Autodesk Fusion 360 part; units mm, degrees
(part 2 of 3)
  line L1099 (31, -19.3397) -> (16, -10.6795)
  line L1100 (63, -19.3397) -> (48, -10.6795)
  line L1101 (31, -19.3397) -> (16, -10.6795)
  line L1102 (-33, -19.3397) -> (-48, -10.6795)
  line L1103 (-1, -36.6603) -> (-1, -19.3397)
  line L1104 (-33, -19.3397) -> (-48, -10.6795)
  line L1105 (-1, -19.3397) -> (-16, -10.6795)
  line L1106 (-33, -19.3397) -> (-48, -10.6795)
  line L1107 (63, -19.3397) -> (48, -10.6795)
  line L1108 (16, -10.6795) -> (1, -19.3397)
  line L1109 (48, -10.6795) -> (33, -19.3397)
  line L1110 (-48, -10.6795) -> (-63, -19.3397)
  line L1111 (48, -10.6795) -> (33, -19.3397)
  line L1112 (-48, -10.6795) -> (-63, -19.3397)
  line L1113 (-33, -36.6603) -> (-33, -19.3397)
  line L1114 (-33, -19.3397) -> (-48, -10.6795)
  line L1115 (-48, -10.6795) -> (-63, -19.3397)
  line L1116 (-31, -19.3397) -> (-31, -36.6603)
  line L1117 (31, -19.3397) -> (16, -10.6795)
  line L1118 (31, -19.3397) -> (16, -10.6795)
  line L1119 (63, -19.3397) -> (48, -10.6795)
  line L1120 (-1, -36.6603) -> (-1, -19.3397)
  line L1121 (48, -10.6795) -> (33, -19.3397)
  line L1122 (48, -10.6795) -> (33, -19.3397)
  line L1123 (-1, -19.3397) -> (-16, -10.6795)
  line L1124 (-48, -10.6795) -> (-63, -19.3397)
  line L1125 (-1, -19.3397) -> (-16, -10.6795)
  line L1126 (-48, -10.6795) -> (-63, -19.3397)
  line L1127 (-1, -36.6603) -> (-1, -19.3397)
  line L1128 (-1, -19.3397) -> (-16, -10.6795)
  line L1129 (-1, -36.6603) -> (-1, -19.3397)
  line L1130 (31, -19.3397) -> (16, -10.6795)
  line L1131 (-1, -19.3397) -> (-16, -10.6795)
  line L1132 (-16, -10.6795) -> (-31, -19.3397)
  line L1133 (-16, -10.6795) -> (-31, -19.3397)
  line L1134 (-33, -36.6603) -> (-33, -19.3397)
  line L1135 (1, -19.3397) -> (1, -36.6603)
  line L1136 (-16, -10.6795) -> (-31, -19.3397)
  line L1137 (1, -19.3397) -> (1, -36.6603)
  line L1138 (1, -19.3397) -> (1, -36.6603)
  line L1139 (-16, -10.6795) -> (-31, -19.3397)
  line L1140 (-16, -10.6795) -> (-31, -19.3397)
  line L1141 (63, -36.6603) -> (63, -19.3397)
  line L1142 (-31, -19.3397) -> (-31, -36.6603)
  line L1143 (-16, -10.6795) -> (-31, -19.3397)
  line L1144 (31, -36.6603) -> (31, -19.3397)
  line L1145 (-16, -10.6795) -> (-31, -19.3397)
  line L1146 (-48, 10.6795) -> (-33, 19.3397)
  line L1147 (33, -19.3397) -> (33, -36.6603)
  line L1148 (32, 17.3205) -> (17, 8.6603)
  line L1149 (33, -19.3397) -> (33, -36.6603)
  line L1150 (-32, -17.3205) -> (-17, -8.6603)
  line L1151 (1, -19.3397) -> (1, -36.6603)
  line L1152 (-32, -17.3205) -> (-17, -8.6603)
  line L1153 (-63, 19.3397) -> (-48, 10.6795)
  line L1154 (31, -36.6603) -> (31, -19.3397)
  line L1155 (31, -36.6603) -> (31, -19.3397)
  line L1156 (31, -36.6603) -> (31, -19.3397)
  line L1157 (-64, 17.3205) -> (-79, 8.6603)
  line L1158 (0, 17.3205) -> (-15, 8.6603)
  line L1159 (1, -19.3397) -> (1, -36.6603)
  line L1160 (-16, -10.6795) -> (-31, -19.3397)
  line L1161 (16, 10.6795) -> (31, 19.3397)
  line L1162 (-16, -10.6795) -> (-31, -19.3397)
  line L1163 (1, -19.3397) -> (1, -36.6603)
  line L1164 (-33, -36.6603) -> (-33, -19.3397)
  line L1165 (-31, -19.3397) -> (-31, -36.6603)
  line L1166 (-16, -10.6795) -> (-31, -19.3397)
  line L1167 (32, 17.3205) -> (17, 8.6603)
  line L1168 (1, -19.3397) -> (1, -36.6603)
  line L1169 (-16, -10.6795) -> (-31, -19.3397)
  line L1170 (-16, -10.6795) -> (-31, -19.3397)
  line L1171 (33, 19.3397) -> (48, 10.6795)
  line L1172 (-64, 17.3205) -> (-79, 8.6603)
  line L1173 (48, 10.6795) -> (63, 19.3397)
  line L1174 (-16, -10.6795) -> (-31, -19.3397)
  line L1175 (-48, 10.6795) -> (-33, 19.3397)
  line L1176 (-16, -10.6795) -> (-31, -19.3397)
  line L1177 (-16, -10.6795) -> (-31, -19.3397)
  line L1178 (-16, 10.6795) -> (-1, 19.3397)
  line L1179 (32, 17.3205) -> (17, 8.6603)
  line L1180 (1, -19.3397) -> (1, -36.6603)
  line L1181 (-16, -10.6795) -> (-31, -19.3397)
  line L1182 (-16, -10.6795) -> (-31, -19.3397)
  line L1183 (32, 17.3205) -> (17, 8.6603)
  line L1184 (-31, -19.3397) -> (-31, -36.6603)
  line L1185 (48, 10.6795) -> (63, 19.3397)
  line L1186 (16, 10.6795) -> (31, 19.3397)
  line L1187 (-16, -10.6795) -> (-31, -19.3397)
  line L1188 (-33, -36.6603) -> (-33, -19.3397)
  line L1189 (-49, 8.6603) -> (-64, 17.3205)
  line L1190 (-32, -17.3205) -> (-17, -8.6603)
  line L1191 (33, -19.3397) -> (33, -36.6603)
  line L1192 (31, -36.6603) -> (31, -19.3397)
  line L1193 (-32, -17.3205) -> (-17, -8.6603)
  line L1194 (1, -19.3397) -> (1, -36.6603)
  line L1195 (-16, -10.6795) -> (-31, -19.3397)
  line L1196 (-16, -10.6795) -> (-31, -19.3397)
  line L1197 (31, -36.6603) -> (31, -19.3397)
  line L1198 (-16, -10.6795) -> (-31, -19.3397)
  line L1199 (-63, 19.3397) -> (-48, 10.6795)
  line L1200 (31, -36.6603) -> (31, -19.3397)
  line L1201 (64, 17.3205) -> (49, 8.6603)
  line L1202 (64, 17.3205) -> (49, 8.6603)
  line L1203 (-32, 17.3205) -> (-47, 8.6603)
  line L1204 (17, -8.6603) -> (32, -17.3205)
  line L1205 (-33, -36.6603) -> (-33, -19.3397)
  line L1206 (31, -36.6603) -> (31, -19.3397)
  line L1207 (-31, -19.3397) -> (-31, -36.6603)
  line L1208 (1, -19.3397) -> (1, -36.6603)
  line L1209 (-32, -17.3205) -> (-17, -8.6603)
  line L1210 (-16, -10.6795) -> (-31, -19.3397)
  line L1211 (-33, -36.6603) -> (-33, -19.3397)
  line L1212 (-33, -36.6603) -> (-33, -19.3397)
  line L1213 (-33, -36.6603) -> (-33, -19.3397)
  line L1214 (-64, 17.3205) -> (-79, 8.6603)
  line L1215 (1, -19.3397) -> (1, -36.6603)
  line L1216 (-16, -10.6795) -> (-31, -19.3397)
  line L1217 (-16, -10.6795) -> (-31, -19.3397)
  line L1218 (31, -36.6603) -> (31, -19.3397)
  line L1219 (31, -36.6603) -> (31, -19.3397)
  line L1220 (-16, -10.6795) -> (-31, -19.3397)
  line L1221 (-64, 17.3205) -> (-79, 8.6603)
  line L1222 (-31, -19.3397) -> (-31, -36.6603)
  line L1223 (47, 8.6603) -> (32, 17.3205)
  line L1224 (1, -19.3397) -> (1, -36.6603)
  line L1225 (-16, -10.6795) -> (-31, -19.3397)
  line L1226 (33, 19.3397) -> (48, 10.6795)
  line L1227 (-49, 8.6603) -> (-64, 17.3205)
  line L1228 (79, 8.6603) -> (64, 17.3205)
  line L1229 (1, -19.3397) -> (1, -36.6603)
  line L1230 (-31, -19.3397) -> (-31, -36.6603)
  line L1231 (63, -36.6603) -> (63, -19.3397)
  line L1232 (33, -19.3397) -> (33, -36.6603)
  line L1233 (79, 8.6603) -> (64, 17.3205)
  line L1234 (-49, 8.6603) -> (-64, 17.3205)
  line L1235 (-49, 8.6603) -> (-64, 17.3205)
  line L1236 (47, 8.6603) -> (32, 17.3205)
  line L1237 (-31, -19.3397) -> (-31, -36.6603)
  line L1238 (79, 8.6603) -> (64, 17.3205)
  line L1239 (79, 8.6603) -> (64, 17.3205)
  line L1240 (47, 8.6603) -> (32, 17.3205)
  line L1241 (-32, -17.3205) -> (-17, -8.6603)
  line L1242 (31, -36.6603) -> (31, -19.3397)
  line L1243 (-17, 8.6603) -> (-32, 17.3205)
  line L1244 (64, 17.3205) -> (49, 8.6603)
  line L1245 (-33, -36.6603) -> (-33, -19.3397)
  line L1246 (31, -36.6603) -> (31, -19.3397)
  line L1247 (47, 8.6603) -> (32, 17.3205)
  line L1248 (31, -36.6603) -> (31, -19.3397)
  line L1249 (-16, -10.6795) -> (-31, -19.3397)
  line L1250 (63, -36.6603) -> (63, -19.3397)
  line L1251 (1, -19.3397) -> (1, -36.6603)
  line L1252 (31, -36.6603) -> (31, -19.3397)
  line L1253 (31, -36.6603) -> (31, -19.3397)
  line L1254 (64, 17.3205) -> (49, 8.6603)
  line L1255 (-1, -19.3397) -> (-16, -10.6795)
  line L1256 (-1, -36.6603) -> (-1, -19.3397)
  line L1257 (-32, 17.3205) -> (-47, 8.6603)
  line L1258 (-31, -19.3397) -> (-31, -36.6603)
  line L1259 (15, 8.6603) -> (0, 17.3205)
  line L1260 (15, 8.6603) -> (0, 17.3205)
  line L1261 (-17, 8.6603) -> (-32, 17.3205)
  line L1262 (-1, -36.6603) -> (-1, -19.3397)
  line L1263 (-1, -19.3397) -> (-16, -10.6795)
  line L1264 (-1, -36.6603) -> (-1, -19.3397)
  line L1265 (17, -8.6603) -> (32, -17.3205)
  line L1266 (-31, 19.3397) -> (-16, 10.6795)
  line L1267 (17, -8.6603) -> (32, -17.3205)
  line L1268 (-32, 17.3205) -> (-47, 8.6603)
  line L1269 (-48, -10.6795) -> (-63, -19.3397)
  line L1270 (17, -8.6603) -> (32, -17.3205)
  line L1271 (-33, -19.3397) -> (-48, -10.6795)
  line L1272 (-33, -36.6603) -> (-33, -19.3397)
  line L1273 (-1, -36.6603) -> (-1, -19.3397)
  line L1274 (-1, -36.6603) -> (-1, -19.3397)
  line L1275 (-31, 19.3397) -> (-16, 10.6795)
  line L1276 (-17, 8.6603) -> (-32, 17.3205)
  line L1277 (17, -8.6603) -> (32, -17.3205)
  line L1278 (-1, -36.6603) -> (-1, -19.3397)
  line L1279 (-31, -19.3397) -> (-31, -36.6603)
  line L1280 (15, 8.6603) -> (0, 17.3205)
  line L1281 (1, 19.3397) -> (16, 10.6795)
  line L1282 (-17, 8.6603) -> (-32, 17.3205)
  line L1283 (-1, -19.3397) -> (-16, -10.6795)
  line L1284 (-1, -36.6603) -> (-1, -19.3397)
  line L1285 (-32, 17.3205) -> (-47, 8.6603)
  line L1286 (17, -8.6603) -> (32, -17.3205)
  line L1287 (15, 8.6603) -> (0, 17.3205)
  line L1288 (-1, -36.6603) -> (-1, -19.3397)
  line L1289 (1, 19.3397) -> (16, 10.6795)
  line L1290 (-1, -36.6603) -> (-1, -19.3397)
  line L1291 (-33, -36.6603) -> (-33, -19.3397)
  line L1292 (-33, -19.3397) -> (-48, -10.6795)
  line L1293 (-48, -10.6795) -> (-63, -19.3397)
  line L1294 (17, -8.6603) -> (32, -17.3205)
  line L1295 (-79, -8.6603) -> (-64, -17.3205)
  line L1296 (-64, -17.3205) -> (-49, -8.6603)
  line L1297 (-64, -17.3205) -> (-49, -8.6603)
  line L1298 (-15, 8.6603) -> (-15, -8.6603)
  line L1299 (-79, -8.6603) -> (-64, -17.3205)
  line L1300 (-15, 8.6603) -> (-15, -8.6603)
  line L1301 (-64, -17.3205) -> (-49, -8.6603)
  line L1302 (-79, -8.6603) -> (-64, -17.3205)
  line L1303 (-79, -8.6603) -> (-64, -17.3205)
  line L1304 (-64, -17.3205) -> (-49, -8.6603)
  line L1305 (-79, 8.6603) -> (-79, -8.6603)
  line L1306 (-79, -8.6603) -> (-64, -17.3205)
  line L1307 (-79, -8.6603) -> (-64, -17.3205)
  line L1308 (-47, 8.6603) -> (-47, -8.6603)
  line L1309 (-49, -8.6603) -> (-49, 8.6603)
  line L1310 (15, -8.6603) -> (15, 8.6603)
  line L1311 (-49, -8.6603) -> (-49, 8.6603)
  line L1312 (-15, 8.6603) -> (-15, -8.6603)
  line L1313 (-17, -8.6603) -> (-17, 8.6603)
  line L1314 (31, -36.6603) -> (31, -19.3397)
  line L1315 (1, -19.3397) -> (1, -36.6603)
  line L1316 (-15, 8.6603) -> (-15, -8.6603)
  line L1317 (1, -19.3397) -> (1, -36.6603)
  line L1318 (-33, -36.6603) -> (-33, -19.3397)
  line L1319 (-16, -10.6795) -> (-31, -19.3397)
  line L1320 (-79, 8.6603) -> (-79, -8.6603)
  line L1321 (-49, -8.6603) -> (-49, 8.6603)
  line L1322 (79, -8.6603) -> (79, 8.6603)
  line L1323 (0, -17.3205) -> (15, -8.6603)
  line L1324 (0, -17.3205) -> (15, -8.6603)
  line L1325 (0, -17.3205) -> (15, -8.6603)
  line L1326 (-31, -19.3397) -> (-31, -36.6603)
  line L1327 (0, -17.3205) -> (15, -8.6603)
  line L1328 (79, -8.6603) -> (79, 8.6603)
  line L1329 (17, 8.6603) -> (17, -8.6603)
  line L1330 (-16, 10.6795) -> (-1, 19.3397)
  line L1331 (47, -8.6603) -> (47, 8.6603)
  line L1332 (-79, 8.6603) -> (-79, -8.6603)
  line L1333 (15, -8.6603) -> (15, 8.6603)
  line L1334 (-47, 8.6603) -> (-47, -8.6603)
  line L1335 (49, 8.6603) -> (49, -8.6603)
  line L1336 (49, 8.6603) -> (49, -8.6603)
  line L1337 (0, -17.3205) -> (15, -8.6603)
  line L1338 (0, -17.3205) -> (15, -8.6603)
  line L1339 (-33, -36.6603) -> (-33, -19.3397)
  line L1340 (0, -17.3205) -> (15, -8.6603)
  line L1341 (0, -17.3205) -> (15, -8.6603)
  line L1342 (63, -36.6603) -> (63, -19.3397)
  line L1343 (-33, -36.6603) -> (-33, -19.3397)
  line L1344 (0, 17.3205) -> (-15, 8.6603)
  line L1345 (-17, -8.6603) -> (-17, 8.6603)
  line L1346 (17, 8.6603) -> (17, -8.6603)
  line L1347 (-32, -17.3205) -> (-17, -8.6603)
  line L1348 (-31, -19.3397) -> (-31, -36.6603)
  line L1349 (-16, -10.6795) -> (-31, -19.3397)
  line L1350 (0, 17.3205) -> (-15, 8.6603)
  line L1351 (-32, -17.3205) -> (-17, -8.6603)
  line L1352 (-16, -10.6795) -> (-31, -19.3397)
  line L1353 (15, -8.6603) -> (15, 8.6603)
  line L1354 (-49, -8.6603) -> (-49, 8.6603)
  line L1355 (47, -8.6603) -> (47, 8.6603)
  line L1356 (17, 8.6603) -> (17, -8.6603)
  line L1357 (-47, 8.6603) -> (-47, -8.6603)
  line L1358 (-16, -10.6795) -> (-31, -19.3397)
  line L1359 (-16, -10.6795) -> (-31, -19.3397)
  line L1360 (0, 17.3205) -> (-15, 8.6603)
  line L1361 (-17, -8.6603) -> (-17, 8.6603)
  line L1362 (-47, 8.6603) -> (-47, -8.6603)
  line L1363 (79, -8.6603) -> (79, 8.6603)
  line L1364 (-31, -19.3397) -> (-31, -36.6603)
  line L1365 (49, 8.6603) -> (49, -8.6603)
  line L1366 (-33, -36.6603) -> (-33, -19.3397)
  line L1367 (47, -8.6603) -> (47, 8.6603)
  line L1368 (-31, -19.3397) -> (-31, -36.6603)
  line L1369 (49, 8.6603) -> (49, -8.6603)
  line L1370 (15, -8.6603) -> (15, 8.6603)
  line L1371 (-31, -19.3397) -> (-31, -36.6603)
  line L1372 (-63, -36.6603) -> (-48, -45.3205)
  line L1373 (-48, -45.3205) -> (-33, -36.6603)
  line L1374 (-31, -36.6603) -> (-16, -45.3205)
  line L1375 (-16, -45.3205) -> (-1, -36.6603)
  line L1376 (1, -36.6603) -> (16, -45.3205)
  line L1377 (16, -45.3205) -> (31, -36.6603)
  line L1378 (48, -45.3205) -> (63, -36.6603)
  line L1379 (33, -36.6603) -> (48, -45.3205)
  line L1380 (-32, 73.3205) -> (-47, 64.6603)
  line L1381 (-47, 64.6603) -> (-47, 47.3397)
  line L1382 (-47, 47.3397) -> (-32, 38.6795)
  line L1383 (-32, 38.6795) -> (-17, 47.3397)
  line L1384 (-17, 47.3397) -> (-17, 64.6603)
  line L1385 (-17, 64.6603) -> (-32, 73.3205)
  line L1386 (0, 38.6795) -> (15, 47.3397)
  line L1387 (-15, 47.3397) -> (0, 38.6795)
  line L1388 (-15, 64.6603) -> (-15, 47.3397)
  line L1389 (0, 73.3205) -> (-15, 64.6603)
  line L1390 (15, 64.6603) -> (0, 73.3205)
  line L1391 (15, 47.3397) -> (15, 64.6603)
  line L1392 (47, 47.3397) -> (47, 64.6603)
  line L1393 (32, 38.6795) -> (47, 47.3397)
  line L1394 (17, 47.3397) -> (32, 38.6795)
  line L1395 (17, 64.6603) -> (17, 47.3397)
  line L1396 (32, 73.3205) -> (17, 64.6603)
  line L1397 (47, 64.6603) -> (32, 73.3205)
  circle A1 centre (0, 0) radius 62
  point P0 (32, 0)
  point P1 (32, 0)
  point P2 (32, 0)
  point P3 (32, 0)
  point P4 (32, 0)
  point P5 (32, 0)
  point P6 (-32, 0)
  point P7 (-32, 0)
  point P8 (-32, 0)
  point P9 (-32, 0)
  point P10 (-32, 0)
  point P11 (-32, 0)
  point P12 (-64, 0)
  point P13 (-64, 0)
  point P14 (-64, 0)
  point P15 (-64, 0)
  point P16 (-64, 0)
  point P17 (-64, 0)
  point P18 (64, 0)
  point P19 (64, 0)
  point P20 (64, 0)
  point P21 (64, 0)
  point P22 (64, 0)
  point P23 (64, 0)
  point P24 (-16, -28)
  point P25 (-16, -28)
  point P26 (-16, -28)
  point P27 (-16, -28)
  point P28 (-16, -28)
  point P29 (-16, -28)
  point P30 (-32, -17.3205)
  point P31 (0, -17.3205)
  point P32 (-16, -28)
  point P33 (-16, -28)
  point P34 (-16, -28)
  point P35 (-16, -28)
  point P36 (-16, -28)
  point P37 (-16, -28)
  point P38 (0, -17.3205)
  point P39 (32, -17.3205)
  point P40 (16, -28)
  point P41 (32, -17.3205)
  point P42 (16, -28)
  point P43 (16, -28)
  point P44 (16, -28)
  point P45 (16, -28)
  point P46 (16, -28)
  point P47 (16, -28)
  point P48 (16, -28)
  point P49 (16, -28)
  point P50 (16, -28)
  point P51 (16, -28)
  point P52 (0, -17.3205)
  point P53 (16, -28)
  point P54 (-49, -8.6603)
  point P55 (-49, -8.6603)
  point P56 (-64, -17.3205)
  point P57 (-47, -8.6603)
  point P58 (-47, -8.6603)
  point P59 (-48, -28)
  point P60 (-48, -28)
  point P61 (-48, -28)
  point P62 (-48, -28)
  point P63 (-48, -28)
  point P64 (-48, -28)
  point P65 (-48, -28)
  point P66 (-48, -28)
  point P67 (-48, -28)
  point P68 (-48, -28)
  point P69 (-48, -28)
  point P70 (-64, -17.3205)
  point P71 (-48, -28)
  point P72 (-32, -56)
  point P73 (-32, -56)
  point P74 (-32, -56)
  point P75 (-64, -56)
  point P76 (-32, -56)
  point P77 (-32, -56)
  point P78 (-32, -56)
  point P79 (32, -56)
  point P80 (32, -56)
  point P81 (32, -56)
  point P82 (32, -56)
  point P83 (0, -56)
  point P84 (0, -56)
  point P85 (32, -56)
  point P86 (0, -56)
  point P87 (32, -56)
  point P88 (0, -56)
  point P89 (0, -56)
  point P90 (0, -56)
  point P91 (32, -73.3205)
  point P92 (0, -73.3205)
  point P93 (-16, -84)
  point P94 (0, -73.3205)
  point P95 (16, -84)
  point P96 (16, -84)
  point P97 (16, -84)
  point P98 (16, -84)
  point P99 (-16, -84)
  point P100 (-16, -84)
  point P101 (-16, -84)
  point P102 (16, -84)
  point P103 (16, -84)
  point P104 (16, -84)
  point P105 (16, -84)
  point P106 (-16, -84)
  point P107 (-16, -84)
  point P108 (16, -84)
  point P109 (16, -84)
  point P110 (16, -84)
  point P111 (32, -73.3205)
  point P112 (-64, -56)
  point P113 (-64, -56)
  point P114 (64, -56)
  point P115 (-64, -56)
  point P116 (-16, -84)
  point P117 (-64, -56)
  point P118 (64, -56)
  point P119 (-16, -84)
  point P120 (-16, -84)
  point P121 (64, -56)
  point P122 (-16, -84)
  point P123 (-16, -84)
  point P124 (-32, -73.3205)
  point P125 (-16, -84)
  point P126 (64, -56)
  point P127 (64, -56)
  point P128 (-64, -56)
  point P129 (64, -56)
  point P130 (-49, -64.6603)
  point P131 (0, -73.3205)
  point P132 (-49, -64.6603)
  point P133 (-48, -84)
  point P134 (-48, -84)
  point P135 (-47, -64.6603)
  point P136 (-47, -64.6603)
  point P137 (-48, -84)
  point P138 (-48, -84)
  point P139 (-48, -84)
  point P140 (-48, -84)
  point P141 (-48, -84)
  point P142 (-48, -84)
  point P143 (16, -84)
  point P144 (-64, -73.3205)
  point P145 (-48, -84)
  point P146 (33, -75.3397)
  point P147 (-64, -73.3205)
  point P148 (-48, -84)
  point P149 (-48, -84)
  point P150 (-48, -84)
  point P151 (-32, 0)
  point P152 (-32, 0)
  point P153 (-17, -8.6603)
  point P154 (-32, 0)
  point P155 (-64, 0)
  point P156 (-32, 0)
  point P157 (-32, 0)
  point P158 (-32, 0)
  point P159 (-47, -8.6603)
  point P160 (32, 0)
  point P161 (17, -8.6603)
  point P162 (32, 0)
  point P163 (32, 0)
  point P164 (32, 0)
  point P165 (15, -8.6603)
  point P166 (32, 0)
  point P167 (32, 0)
  point P168 (47, -8.6603)
  point P169 (-15, -8.6603)
  point P170 (0, -56)
  point P171 (-32, -56)
  point P172 (-32, -56)
  point P173 (0, -56)
  point P174 (-32, -56)
  point P175 (32, -56)
  point P176 (0, -56)
  point P177 (-32, -56)
  point P178 (-64, -56)
  point P179 (32, -56)
  point P180 (-32, -56)
  point P181 (-32, -56)
  point P182 (32, -56)
  point P183 (32, -56)
  point P184 (0, -56)
  point P185 (0, -56)
  point P186 (32, -56)
  point P187 (0, -56)
  point P188 (32, -56)
  point P189 (32, -17.3205)
  point P190 (0, -17.3205)
  point P191 (-16, -28)
  point P192 (0, -17.3205)
  point P193 (16, -28)
  point P194 (16, -28)
  point P195 (16, -28)
  point P196 (16, -28)
  point P197 (-16, -28)
  point P198 (-16, -28)
  point P199 (-16, -28)
  point P200 (16, -28)
  point P201 (16, -28)
  point P202 (16, -28)
  point P203 (16, -28)
  point P204 (-16, -28)
  point P205 (-16, -28)
  point P206 (16, -28)
  point P207 (16, -28)
  point P208 (16, -28)
  point P209 (32, -17.3205)
  point P210 (-48, -84)
  point P211 (33, -75.3397)
  point P212 (-48, -84)
  point P213 (-48, -84)
  point P214 (-48, -84)
  point P215 (16, -84)
  point P216 (-48, -84)
  point P217 (-64, -73.3205)
  point P218 (-64, -73.3205)
  point P219 (-64, 0)
  point P220 (-64, 0)
  point P221 (-79, -8.6603)
  point P222 (49, -8.6603)
  point P223 (79, -8.6603)
  point P224 (64, 0)
  point P225 (-64, 0)
  point P226 (-16, -28)
  point P227 (-64, 0)
  point P228 (64, 0)
  point P229 (-16, -28)
  point P230 (-16, -28)
  point P231 (-49, -8.6603)
  point P232 (64, 0)
  point P233 (-16, -28)
  point P234 (-16, -28)
  point P235 (-32, -17.3205)
  point P236 (-16, -28)
  point P237 (64, 0)
  point P238 (64, 0)
  point P239 (-64, 0)
  point P240 (64, 0)
  point P241 (-49, -8.6603)
  point P242 (0, -17.3205)
  point P243 (-49, -8.6603)
  point P244 (-48, -28)
  point P245 (-48, -28)
  point P246 (-47, -8.6603)
  point P247 (-47, -8.6603)
  point P248 (-48, -28)
  point P249 (-48, -28)
  point P250 (-48, -28)
  point P251 (-48, -28)
  point P252 (-48, -28)
  point P253 (-48, -28)
  point P254 (16, -28)
  point P255 (-64, -17.3205)
  point P256 (-48, -28)
  point P257 (-64, -17.3205)
  point P258 (-48, -28)
  point P259 (-48, -28)
  point P260 (-48, -28)
  point P261 (16, -84)
  point P262 (32, -73.3205)
  point P263 (16, -84)
  point P264 (16, -84)
  point P265 (-16, -84)
  point P266 (16, -84)
  point P267 (-16, -84)
  point P268 (16, -84)
  point P269 (-16, -84)
  point P270 (-16, -84)
  point P271 (16, -84)
  point P272 (16, -84)
  point P273 (-64, -56)
  point P274 (16, -84)
  point P275 (16, -84)
  point P276 (64, -56)
  point P277 (16, -84)
  point P278 (32, -73.3205)
  point P279 (-64, -56)
  point P280 (0, -73.3205)
  point P281 (-16, -84)
  point P282 (-64, -56)
  point P283 (-16, -84)
  point P284 (0, -73.3205)
  point P285 (-16, -84)
  point P286 (16, -84)
  point P287 (-64, -56)
  point P288 (64, -56)
  point P289 (-16, -84)
  point P290 (-48, -84)
  point P291 (-48, -84)
  point P292 (64, -56)
  point P293 (-64, -56)
  point P294 (-16, -84)
  point P295 (-48, -84)
  point P296 (-16, -84)
  point P297 (-32, -73.3205)
  point P298 (-49, -64.6603)
  point P299 (-47, -64.6603)
  point P300 (-48, -84)
  point P301 (64, -56)
  point P302 (64, -56)
  point P303 (64, -56)
  point P304 (0, -73.3205)
  point P305 (-49, -64.6603)
  point P306 (-48, -84)
  point P307 (-16, -84)
  point P308 (-16, -84)
  point P309 (-47, -64.6603)
  point P310 (-48, -84)
  point P311 (-48, -84)
  point P312 (-17, -8.6603)
  point P313 (-47, -8.6603)
  point P314 (17, -8.6603)
  point P315 (15, -8.6603)
  point P316 (47, -8.6603)
  point P317 (-15, -8.6603)
  point P318 (0, -56)
  point P319 (-32, -56)
  point P320 (-32, -56)
  point P321 (0, -56)
  point P322 (-32, -56)
  point P323 (32, -56)
  point P324 (0, -56)
  point P325 (-32, -56)
  point P326 (-64, -56)
  point P327 (32, -56)
  point P328 (-32, -56)
  point P329 (-32, -56)
  point P330 (32, -56)
  point P331 (32, -56)
  point P332 (0, -56)
  point P333 (0, -56)
  point P334 (32, -56)
  point P335 (0, -56)
  point P336 (32, -56)
  point P337 (32, -17.3205)
  point P338 (0, -17.3205)
  point P339 (-16, -28)
  point P340 (0, -17.3205)
  point P341 (16, -28)
  point P342 (16, -28)
  point P343 (16, -28)
  point P344 (16, -28)
  point P345 (-16, -28)
  point P346 (-16, -28)
  point P347 (-16, -28)
  point P348 (16, -28)
  point P349 (16, -28)
  point P350 (16, -28)
  point P351 (16, -28)
  point P352 (-16, -28)
  point P353 (-16, -28)
  point P354 (16, -28)
  point P355 (16, -28)
  point P356 (16, -28)
  point P357 (32, -17.3205)
  point P358 (-32, -56)
  point P359 (-47, -8.6603)
  point P360 (48, -66.6795)
  point P361 (-48, -66.6795)
  point P362 (-17, -8.6603)
  point P363 (0, -56)
  point P364 (15, -8.6603)
  point P365 (47, -8.6603)
  point P366 (-15, -8.6603)
  point P367 (17, -8.6603)
  point P368 (0, -56)
  point P369 (-32, -56)
  point P370 (32, -56)
  point P371 (32, -56)
  point P372 (32, -56)
  point P373 (0, -56)
  point P374 (-32, -56)
  point P375 (-32, -56)
  point P376 (-64, -56)
  point P377 (-32, -56)
  point P378 (-32, -56)
  point P379 (32, -56)
  point P380 (0, -56)
  point P381 (0, -56)
  point P382 (32, -56)
  point P383 (32, -56)
  point P384 (0, -56)
  point P385 (32, -17.3205)
  point P386 (-79, -8.6603)
  point P387 (49, -8.6603)
  point P388 (79, -8.6603)
  point P389 (-16, -28)
  point P390 (-16, -28)
  point P391 (-16, -28)
  point P392 (-49, -8.6603)
  point P393 (-16, -28)
  point P394 (-16, -28)
  point P395 (-32, -17.3205)
  point P396 (-16, -28)
  point P397 (-49, -8.6603)
  point P398 (0, -17.3205)
  point P399 (-49, -8.6603)
  point P400 (-48, -28)
  point P401 (-48, -28)
  point P402 (-47, -8.6603)
  point P403 (-47, -8.6603)
  point P404 (-48, -28)
  point P405 (-48, -28)
  point P406 (-48, -28)
  point P407 (-48, -28)
  point P408 (-48, -28)
  point P409 (-48, -28)
  point P410 (16, -28)
  point P411 (-64, -17.3205)
  point P412 (-48, -28)
  point P413 (-64, -17.3205)
  point P414 (-48, -28)
  point P415 (-48, -28)
  point P416 (-48, -28)
  point P417 (32, -17.3205)
  point P418 (16, -28)
  point P419 (-16, -28)
  point P420 (-16, -28)
  point P421 (16, -28)
  point P422 (-16, -28)
  point P423 (16, -28)
  point P424 (16, -28)
  point P425 (-16, -28)
  point P426 (16, -28)
  point P427 (16, -28)
  point P428 (16, -28)
  point P429 (0, -17.3205)
  point P430 (0, -17.3205)
  point P431 (16, -28)
  point P432 (16, -28)
  point P433 (-16, -28)
  point P434 (-16, -28)
  point P435 (16, -28)
  point P436 (16, -28)
  point P437 (48, -66.6795)
  point P438 (-48, -66.6795)
  point P439 (-16, -28)
  point P440 (-49, -8.6603)
  point P441 (-79, -8.6603)
  point P442 (-16, -28)
  point P443 (79, -8.6603)
  point P444 (-16, -28)
  point P445 (-16, -28)
  point P446 (49, -8.6603)
  point P447 (-16, -28)
  point P448 (-32, -17.3205)
  point P449 (-16, -28)
  point P450 (16, -66.6795)
  point P451 (16, -66.6795)
  point P452 (16, -66.6795)
  point P453 (16, -66.6795)
  point P454 (-16, -66.6795)
  point P455 (-64, -56)
  point P456 (64, -56)
  point P457 (-16, -66.6795)
  point P458 (-64, -56)
  point P459 (-64, -56)
  point P460 (-16, -66.6795)
  point P461 (-64, -56)
  point P462 (-16, -66.6795)
  point P463 (64, -56)
  point P464 (-48, -66.6795)
  point P465 (64, -56)
  point P466 (-64, -56)
  point P467 (-48, -66.6795)
  point P468 (-49, -64.6603)
  point P469 (-47, -64.6603)
  point P470 (64, -56)
  point P471 (64, -56)
  point P472 (48, -66.6795)
  point P473 (64, -56)
  point P474 (-49, -64.6603)
  point P475 (-47, -64.6603)
  point P476 (-48, -66.6795)
  point P477 (-48, -66.6795)
  point P478 (-47, -64.6603)
  point P479 (-49, -64.6603)
  point P480 (-47, -8.6603)
  point P481 (16, -28)
  point P482 (-48, -28)
  point P483 (-48, -28)
  point P484 (-49, -8.6603)
  point P485 (0, -17.3205)
  point P486 (-48, -28)
  point P487 (-48, -28)
  point P488 (-64, -17.3205)
  point P489 (-48, -28)
  point P490 (-48, -28)
  point P491 (-47, -8.6603)
  point P492 (-48, -28)
  point P493 (-48, -28)
  point P494 (-49, -8.6603)
  point P495 (-48, -28)
  point P496 (-48, -28)
  point P497 (-48, -28)
  point P498 (-48, -28)
  point P499 (-64, -17.3205)
  point P500 (16, -66.6795)
  point P501 (16, -66.6795)
  point P502 (-16, -66.6795)
  point P503 (-16, -66.6795)
  point P504 (-16, -66.6795)
  point P505 (-64, -56)
  point P506 (-64, -56)
  point P507 (16, -66.6795)
  point P508 (-16, -66.6795)
  point P509 (-48, -66.6795)
  point P510 (16, -66.6795)
  point P511 (-64, -56)
  point P512 (-64, -56)
  point P513 (64, -56)
  point P514 (64, -56)
  point P515 (64, -56)
  point P516 (-64, -56)
  point P517 (-48, -66.6795)
  point P518 (48, -66.6795)
  point P519 (64, -56)
  point P520 (-47, -64.6603)
  point P521 (64, -56)
  point P522 (64, -56)
  point P523 (-49, -64.6603)
  point P524 (0, 17.3205)
  point P525 (32, 17.3205)
  point P526 (-32, 17.3205)
  point P527 (-32, 17.3205)
  point P528 (32, 17.3205)
  point P529 (0, 17.3205)
  point P530 (-16, 28)
  point P531 (16, 28)
  point P532 (16, 28)
  point P533 (16, 28)
  point P534 (16, 28)
  point P535 (-16, 28)
  point P536 (-16, 28)
  point P537 (-16, 28)
  point P538 (16, 28)
  point P539 (16, 28)
  point P540 (16, 28)
  point P541 (16, 28)
  point P542 (-16, 28)
  point P543 (-16, 28)
  point P544 (16, 28)
  point P545 (16, 28)
  point P546 (16, 28)
  point P547 (0, 17.3205)
  point P548 (32, 17.3205)
  point P549 (-32, 17.3205)
  point P550 (63, 19.3397)
  point P551 (32, 17.3205)
  point P552 (0, 17.3205)
  point P553 (-32, 17.3205)
  point P554 (-16, 28)
  point P555 (-16, 28)
  point P556 (-16, 28)
  point P557 (-16, 28)
  point P558 (-16, 28)
  point P559 (-16, 28)
  point P560 (-48, 28)
  point P561 (-48, 28)
  point P562 (-48, 28)
  point P563 (-48, 28)
  point P564 (-48, 28)
  point P565 (-48, 28)
  point P566 (-48, 28)
  point P567 (-48, 28)
  point P568 (16, 28)
  point P569 (-48, 28)
  point P570 (-48, 28)
  point P571 (-48, 28)
  point P572 (-48, 28)
  point P573 (16, 28)
  point P574 (-16, 28)
  point P575 (-16, 28)
  point P576 (16, 28)
  point P577 (-16, 28)
  point P578 (16, 28)
  point P579 (33, 19.3397)
  point P580 (16, 28)
  point P581 (-16, 28)
  point P582 (16, 28)
  point P583 (16, 28)
  point P584 (16, 28)
  point P585 (16, 28)
  point P586 (16, 28)
  point P587 (-16, 28)
  point P588 (-16, 28)
  point P589 (16, 28)
  point P590 (16, 28)
  point P591 (-16, 28)
  point P592 (-16, 28)
  point P593 (-16, 28)
  point P594 (-16, 28)
  point P595 (-16, 28)
  point P596 (-16, 28)
  point P597 (64, 17.3205)
  point P598 (64, 17.3205)
  point P599 (-64, 17.3205)
  point P600 (-64, 17.3205)
  point P601 (0, 17.3205)
  point P602 (-32, 17.3205)
  point P603 (-32, 17.3205)
  point P604 (32, 17.3205)
  point P605 (63, 19.3397)
  point P606 (16, 28)
  point P607 (-48, 28)
  point P608 (-48, 28)
  point P609 (-48, 28)
  point P610 (-48, 28)
  point P611 (-48, 28)
  point P612 (-48, 28)
  point P613 (-48, 28)
  point P614 (-48, 28)
  point P615 (-48, 28)
  point P616 (-48, 28)
  point P617 (-48, 28)
  point P618 (-48, 28)
  point P619 (64, 17.3205)
  point P620 (-64, 17.3205)
  point P621 (64, 17.3205)
  point P622 (-64, 17.3205)
  point P623 (16, 28)
  point P624 (16, 28)
  point P625 (33, 19.3397)
  point P626 (16, 28)
  point P627 (16, 28)
  point P628 (-16, 28)
  point P629 (16, 28)
  point P630 (-16, 28)
  point P631 (16, 28)
  point P632 (-16, 28)
  point P633 (16, 28)
  point P634 (16, 28)
  point P635 (0, 17.3205)
  point P636 (32, 17.3205)
  point P637 (-16, 28)
  point P638 (16, 28)
  point P639 (-16, 28)
  point P640 (16, 28)
  point P641 (16, 28)
  point P642 (-16, 28)
  point P643 (-32, 17.3205)
  point P644 (63, 19.3397)
  point P645 (32, 17.3205)
  point P646 (32, 17.3205)
  point P647 (0, 17.3205)
  point P648 (0, 17.3205)
  point P649 (-16, 28)
  point P650 (-16, 28)
  point P651 (-16, 28)
  point P652 (-32, 17.3205)
  point P653 (-48, 28)
  point P654 (-16, 28)
  point P655 (-48, 28)
  point P656 (-16, 28)
  point P657 (-16, 28)
  point P658 (-48, 28)
  point P659 (-48, 28)
  point P660 (-48, 28)
  point P661 (-48, 28)
  point P662 (-48, 28)
  point P663 (16, 28)
  point P664 (-48, 28)
  point P665 (-48, 28)
  point P666 (-48, 28)
  point P667 (-48, 28)
  point P668 (-48, 28)
  point P669 (-48, 28)
  point P670 (-48, 28)
  point P671 (-48, 28)
  point P672 (-48, 28)
  point P673 (-48, 28)
  point P674 (-48, 28)
  point P675 (-48, 28)
  point P676 (64, 17.3205)
  point P677 (-64, 17.3205)
  point P678 (-16, 28)
  point P679 (16, 28)
  point P680 (16, 28)
  point P681 (16, 28)
  point P682 (-16, 28)
  point P683 (-48, 28)
  point P684 (-48, 28)
  point P685 (16, 28)
  point P686 (16, 28)
  point P687 (16, 28)
  point P688 (-16, 28)
  point P689 (-16, 28)
  point P690 (33, 19.3397)
  point P691 (-16, 28)
  point P692 (16, 28)
  point P693 (-48, 28)
  point P694 (16, 28)
  point P695 (16, 28)
  point P696 (-16, 28)
  point P697 (16, 28)
  point P698 (16, 28)
  point P699 (-16, 28)
  point P700 (-64, 17.3205)
  point P701 (64, 17.3205)
  point P702 (-64, 17.3205)
  point P703 (-16, 28)
  point P704 (64, 17.3205)
  point P705 (-16, 28)
  point P706 (-16, 28)
  point P707 (-16, 28)
  point P708 (-16, 28)
  point P709 (16, 28)
  point P710 (-48, 28)
  point P711 (-48, 28)
  point P712 (64, 17.3205)
  point P713 (-64, 17.3205)
  point P714 (-32, 0)
  point P715 (-32, 0)
  point P716 (-32, 0)
  point P717 (-64, 0)
  point P718 (-32, 0)
  point P719 (-32, 0)
  point P720 (-32, 0)
  point P721 (32, 0)
  point P722 (32, 0)
  point P723 (32, 0)
  point P724 (32, 0)
  point P725 (32, 0)
  point P726 (32, 0)
  point P727 (32, -17.3205)
  point P728 (0, -17.3205)
  point P729 (0, -17.3205)
  point P730 (32, -17.3205)
  point P731 (-32, 0)
  point P732 (-64, 0)
  point P733 (-47, -8.6603)
  point P734 (32, 0)
  point P735 (32, 0)
  point P736 (32, 0)
  point P737 (-17, -8.6603)
  point P738 (-32, 0)
  point P739 (15, -8.6603)
  point P740 (32, 0)
  point P741 (47, -8.6603)
  point P742 (-32, 0)
  point P743 (-32, 0)
  point P744 (32, 0)
  point P745 (-32, 0)
  point P746 (-15, -8.6603)
  point P747 (17, -8.6603)
  point P748 (-32, 0)
  point P749 (32, 0)
  point P750 (32, -17.3205)
  point P751 (-64, 0)
  point P752 (-64, 0)
  point P753 (64, 0)
  point P754 (-64, 0)
  point P755 (-64, 0)
  point P756 (64, 0)
  point P757 (64, 0)
  point P758 (-32, -17.3205)
  point P759 (64, 0)
  point P760 (64, 0)
  point P761 (-64, 0)
  point P762 (64, 0)
  point P763 (-49, -8.6603)
  point P764 (0, -17.3205)
  point P765 (-49, -8.6603)
  point P766 (-47, -8.6603)
  point P767 (-47, -8.6603)
  point P768 (-64, -17.3205)
  point P769 (33, -19.3397)
  point P770 (-64, -17.3205)
  point P771 (32, -17.3205)
  point P772 (0, -17.3205)
  point P773 (0, -17.3205)
  point P774 (64, 0)
  point P775 (-64, 0)
  point P776 (64, 0)
  point P777 (-49, -8.6603)
  point P778 (-79, -8.6603)
  point P779 (79, -8.6603)
  point P780 (-64, 0)
  point P781 (64, 0)
  point P782 (64, 0)
  point P783 (64, 0)
  point P784 (-64, 0)
  point P785 (49, -8.6603)
  point P786 (-64, 0)
  point P787 (-64, 0)
  point P788 (-32, -17.3205)
  point P789 (64, 0)
  point P790 (47, -8.6603)
  point P791 (-47, -8.6603)
  point P792 (17, -8.6603)
  point P793 (15, -8.6603)
  point P794 (-15, -8.6603)
  point P795 (-17, -8.6603)
  point P796 (-47, -8.6603)
  point P797 (-49, -8.6603)
  point P798 (0, -17.3205)
  point P799 (-64, -17.3205)
  point P800 (-47, -8.6603)
  point P801 (-49, -8.6603)
  point P802 (-64, -17.3205)
  point P803 (33, -19.3397)
  point P804 (32, -17.3205)
  point P805 (0, -17.3205)
  point P806 (32, -17.3205)
  point P807 (0, -17.3205)
  point P808 (17, -8.6603)
  point P809 (-17, -8.6603)
  point P810 (47, -8.6603)
  point P811 (15, -8.6603)
  point P812 (-15, -8.6603)
  point P813 (-47, -8.6603)
  point P814 (-79, -8.6603)
  point P815 (32, -17.3205)
  point P816 (-47, -8.6603)
  point P817 (49, -8.6603)
  point P818 (-32, -17.3205)
  point P819 (79, -8.6603)
  point P820 (-49, -8.6603)
  point P821 (0, -17.3205)
  point P822 (-49, -8.6603)
  point P823 (-49, -8.6603)
  point P824 (-47, -8.6603)
  point P825 (-64, -17.3205)
  point P826 (-49, -8.6603)
  point P827 (-47, -8.6603)
  point P828 (-64, -17.3205)
  point P829 (0, -17.3205)
  point P830 (-64, -17.3205)
  point P831 (33, -19.3397)
  point P832 (33, -19.3397)
  point P833 (0, -17.3205)
  point P834 (-64, -17.3205)
  point P835 (0, -17.3205)
  point P836 (32, -17.3205)
  point P837 (79, -8.6603)
  point P838 (-49, -8.6603)
  point P839 (-32, -17.3205)
  point P840 (-79, -8.6603)
  point P841 (49, -8.6603)
  point P842 (-47, -8.6603)
  point P843 (-49, -8.6603)
  point P844 (-31, 19.3397)
  point P845 (-31, 19.3397)
  point P846 (-1, 19.3397)
  point P847 (64, 17.3205)
  point P848 (-1, 19.3397)
  point P849 (33, 19.3397)
  point P850 (31, 19.3397)
  point P851 (-64, 17.3205)
  point P852 (64, 17.3205)
  point P853 (-64, 17.3205)
  point P854 (-32, 17.3205)
  point P855 (63, 19.3397)
  point P856 (33, 19.3397)
  point P857 (31, 19.3397)
  point P858 (1, 19.3397)
  point P859 (-32, 17.3205)
  point P860 (32, 17.3205)
  point P861 (0, 17.3205)
  point P862 (-31, 19.3397)
  point P863 (0, 17.3205)
  point P864 (1, 19.3397)
  point P865 (-32, 17.3205)
  point P866 (32, 17.3205)
  point P867 (-32, 17.3205)
  point P868 (-1, 19.3397)
  point P869 (32, 17.3205)
  point P870 (1, 19.3397)
  point P871 (31, 19.3397)
  point P872 (31, 19.3397)
  point P873 (0, 17.3205)
  point P874 (-1, 19.3397)
  point P875 (-31, 19.3397)
  point P876 (-31, 19.3397)
  point P877 (-1, 19.3397)
  point P878 (-1, 19.3397)
  point P879 (-32, 17.3205)
  point P880 (32, 17.3205)
  point P881 (0, 17.3205)
  point P882 (-31, 19.3397)
  point P883 (31, 19.3397)
  point P884 (63, 19.3397)
  point P885 (-63, 19.3397)
  point P886 (33, 19.3397)
  point P887 (-32, 17.3205)
  point P888 (-33, 19.3397)
  point P889 (63, 19.3397)
  point P890 (-33, 19.3397)
  point P891 (-63, 19.3397)
  point P892 (32, 17.3205)
  point P893 (0, 17.3205)
  point P894 (1, 19.3397)
  point P895 (-33, 19.3397)
  point P896 (-63, 19.3397)
  point P897 (1, 19.3397)
  point P898 (-33, 19.3397)
  point P899 (-31, 19.3397)
  point P900 (1, 19.3397)
  point P901 (31, 19.3397)
  point P902 (31, 19.3397)
  point P903 (-33, 19.3397)
  point P904 (1, 19.3397)
  point P905 (1, 19.3397)
  point P906 (-31, 19.3397)
  point P907 (0, 17.3205)
  point P908 (-63, 19.3397)
  point P909 (31, 19.3397)
  point P910 (-33, 19.3397)
  point P911 (-33, 19.3397)
  point P912 (63, 19.3397)
  point P913 (1, 19.3397)
  point P914 (-63, 19.3397)
  point P915 (-64, 17.3205)
  point P916 (-64, 17.3205)
  point P917 (-1, 19.3397)
  point P918 (-63, 19.3397)
  point P919 (64, 17.3205)
  point P920 (-1, 19.3397)
  point P921 (-1, 19.3397)
  point P922 (-63, 19.3397)
  point P923 (64, 17.3205)
  point P924 (33, 19.3397)
  point P925 (1, 19.3397)
  point P926 (32, 17.3205)
  point P927 (-63, 19.3397)
  point P928 (32, 17.3205)
  point P929 (-33, 19.3397)
  point P930 (33, 19.3397)
  point P931 (-33, 19.3397)
  point P932 (-33, 19.3397)
  point P933 (-31, 19.3397)
  point P934 (-1, 19.3397)
  point P935 (32, 17.3205)
  point P936 (-32, 17.3205)
  point P937 (-31, 19.3397)
  point P938 (-63, 19.3397)
  point P939 (63, 19.3397)
  point P940 (0, 17.3205)
  point P941 (-33, 19.3397)
  point P942 (-63, 19.3397)
  point P943 (31, 19.3397)
  point P944 (-1, 19.3397)
  point P945 (-32, 17.3205)
  point P946 (31, 19.3397)
  point P947 (0, 17.3205)
  point P948 (-33, 19.3397)
  point P949 (-31, 19.3397)
  point P950 (-63, 19.3397)
  point P951 (63, 19.3397)
  point P952 (1, 19.3397)
  point P953 (-64, 17.3205)
  point P954 (-31, 19.3397)
  point P955 (-33, 19.3397)
  point P956 (-63, 19.3397)
  point P957 (-1, 19.3397)
  point P958 (1, 19.3397)
  point P959 (-33, 19.3397)
  point P960 (63, 19.3397)
  point P961 (-31, 19.3397)
  point P962 (1, 19.3397)
  point P963 (31, 19.3397)
  point P964 (-63, 19.3397)
  point P965 (-33, 19.3397)
  point P966 (31, 19.3397)
  point P967 (-1, 19.3397)
  point P968 (1, 19.3397)
  point P969 (-63, 19.3397)
  point P970 (-63, 19.3397)
  point P971 (64, 17.3205)
  point P972 (31, 19.3397)
  point P973 (-31, 19.3397)
  point P974 (1, 19.3397)
  point P975 (-31, 19.3397)
  point P976 (64, 17.3205)
  point P977 (64, 17.3205)
  point P978 (-1, 19.3397)
  point P979 (-1, 19.3397)
  point P980 (-64, 17.3205)
  point P981 (-64, 17.3205)
  point P982 (33, 19.3397)
  point P983 (33, 19.3397)
  point P984 (31, 19.3397)
  point P985 (31, 19.3397)
  point P986 (-64, 17.3205)
  point P987 (64, 17.3205)
  point P988 (-32, 0)
  point P989 (-32, 0)
  point P990 (-32, 0)
  point P991 (-64, 0)
  point P992 (-32, 0)
  point P993 (-32, 0)
  point P994 (-32, 0)
  point P995 (32, 0)
  point P996 (32, 0)
  point P997 (32, 0)
  point P998 (32, 0)
  point P999 (32, 0)
  point P1000 (32, 0)
  point P1001 (32, -17.3205)
  point P1002 (0, -17.3205)
  point P1003 (-16, -28)
  point P1004 (0, -17.3205)
  point P1005 (16, -28)
  point P1006 (16, -28)
  point P1007 (16, -28)
  point P1008 (16, -28)
  point P1009 (-16, -28)
  point P1010 (-16, -28)
  point P1011 (-16, -28)
  point P1012 (16, -28)
  point P1013 (16, -28)
  point P1014 (16, -28)
  point P1015 (16, -28)
  point P1016 (-16, -28)
  point P1017 (-16, -28)
  point P1018 (16, -28)
  point P1019 (16, -28)
  point P1020 (16, -28)
  point P1021 (32, -17.3205)
  point P1022 (-32, 0)
  point P1023 (-64, 0)
  point P1024 (-47, -8.6603)
  point P1025 (32, 0)
  point P1026 (32, 0)
  point P1027 (32, 0)
  point P1028 (-17, -8.6603)
  point P1029 (-32, 0)
  point P1030 (15, -8.6603)
  point P1031 (32, 0)
  point P1032 (47, -8.6603)
  point P1033 (-32, 0)
  point P1034 (-32, 0)
  point P1035 (32, 0)
  point P1036 (-32, 0)
  point P1037 (-15, -8.6603)
  point P1038 (17, -8.6603)
  point P1039 (-32, 0)
  point P1040 (32, 0)
  point P1041 (32, -17.3205)
  point P1042 (-64, 0)
  point P1043 (-64, 0)
  point P1044 (64, 0)
  point P1045 (-64, 0)
  point P1046 (-16, -28)
  point P1047 (-64, 0)
  point P1048 (64, 0)
  point P1049 (-16, -28)
  point P1050 (-16, -28)
  point P1051 (64, 0)
  point P1052 (-16, -28)
  point P1053 (-16, -28)
  point P1054 (-32, -17.3205)
  point P1055 (-16, -28)
  point P1056 (64, 0)
  point P1057 (64, 0)
  point P1058 (-64, 0)
  point P1059 (64, 0)
  point P1060 (-49, -8.6603)
  point P1061 (0, -17.3205)
  point P1062 (-49, -8.6603)
  point P1063 (-48, -28)
  point P1064 (-48, -28)
  point P1065 (-47, -8.6603)
  point P1066 (-47, -8.6603)
  point P1067 (-48, -28)
  point P1068 (-48, -28)
  point P1069 (-48, -28)
  point P1070 (-48, -28)
  point P1071 (-48, -28)
  point P1072 (-48, -28)
  point P1073 (16, -28)
  point P1074 (-64, -17.3205)
  point P1075 (-48, -28)
  point P1076 (-64, -17.3205)
  point P1077 (-48, -28)
  point P1078 (-48, -28)
  point P1079 (-48, -28)
  point P1080 (32, -17.3205)
  point P1081 (16, -28)
  point P1082 (-16, -28)
  point P1083 (-16, -28)
  point P1084 (16, -28)
  point P1085 (-16, -28)
  point P1086 (16, -28)
  point P1087 (16, -28)
  point P1088 (-16, -28)
  point P1089 (16, -28)
  point P1090 (16, -28)
  point P1091 (16, -28)
  point P1092 (0, -17.3205)
  point P1093 (0, -17.3205)
  point P1094 (16, -28)
  point P1095 (16, -28)
  point P1096 (-16, -28)
  point P1097 (-16, -28)
  point P1098 (16, -28)
  point P1099 (16, -28)
  point P1100 (-16, -28)
  point P1101 (64, 0)
  point P1102 (-64, 0)
  point P1103 (64, 0)
  point P1104 (-49, -8.6603)
  point P1105 (-79, -8.6603)
  point P1106 (-16, -28)
  point P1107 (79, -8.6603)
  point P1108 (-64, 0)
  point P1109 (64, 0)
  point P1110 (64, 0)
  point P1111 (-16, -28)
  point P1112 (64, 0)
  point P1113 (-16, -28)
  point P1114 (-64, 0)
  point P1115 (49, -8.6603)
  point P1116 (-64, 0)
  point P1117 (-64, 0)
  point P1118 (-16, -28)
  point P1119 (-32, -17.3205)
  point P1120 (-16, -28)
  point P1121 (64, 0)
  point P1122 (47, -8.6603)
  point P1123 (-47, -8.6603)
  point P1124 (17, -8.6603)
  point P1125 (15, -8.6603)
  point P1126 (-15, -8.6603)
  point P1127 (-17, -8.6603)
  point P1128 (-47, -8.6603)
  point P1129 (16, -28)
  point P1130 (-48, -28)
  point P1131 (-48, -28)
  point P1132 (-49, -8.6603)
  point P1133 (0, -17.3205)
  point P1134 (-48, -28)
  point P1135 (-48, -28)
  point P1136 (-64, -17.3205)
  point P1137 (-48, -28)
  point P1138 (-48, -28)
  point P1139 (-47, -8.6603)
  point P1140 (-48, -28)
  point P1141 (-48, -28)
  point P1142 (-49, -8.6603)
  point P1143 (-48, -28)
  point P1144 (-48, -28)
  point P1145 (-48, -28)
  point P1146 (-48, -28)
  point P1147 (-64, -17.3205)
  point P1148 (16, -28)
  point P1149 (32, -17.3205)
  point P1150 (0, -17.3205)
  point P1151 (16, -28)
  point P1152 (16, -28)
  point P1153 (16, -28)
  point P1154 (-16, -28)
  point P1155 (16, -28)
  point P1156 (-16, -28)
  point P1157 (16, -28)
  point P1158 (-16, -28)
  point P1159 (16, -28)
  point P1160 (16, -28)
  point P1161 (32, -17.3205)
  point P1162 (-16, -28)
  point P1163 (0, -17.3205)
  point P1164 (16, -28)
  point P1165 (-16, -28)
  point P1166 (16, -28)
  point P1167 (16, -28)
  point P1168 (-16, -28)
  point P1169 (17, -8.6603)
  point P1170 (-17, -8.6603)
  point P1171 (47, -8.6603)
  point P1172 (15, -8.6603)
  point P1173 (-15, -8.6603)
  point P1174 (-47, -8.6603)
  point P1175 (-79, -8.6603)
  point P1176 (32, -17.3205)
  point P1177 (-16, -28)
  point P1178 (-47, -8.6603)
  point P1179 (-16, -28)
  point P1180 (49, -8.6603)
  point P1181 (-32, -17.3205)
  point P1182 (79, -8.6603)
  point P1183 (-16, -28)
  point P1184 (-49, -8.6603)
  point P1185 (0, -17.3205)
  point P1186 (-48, -28)
  point P1187 (-16, -28)
  point P1188 (-48, -28)
  point P1189 (-16, -28)
  point P1190 (-49, -8.6603)
  point P1191 (-16, -28)
  point P1192 (-49, -8.6603)
  point P1193 (-48, -28)
  point P1194 (-48, -28)
  point P1195 (-48, -28)
  point P1196 (-47, -8.6603)
  point P1197 (-48, -28)
  point P1198 (-64, -17.3205)
  point P1199 (-48, -28)
  point P1200 (16, -28)
  point P1201 (-48, -28)
  point P1202 (-48, -28)
  point P1203 (-48, -28)
  point P1204 (-49, -8.6603)
  point P1205 (-48, -28)
  point P1206 (-48, -28)
  point P1207 (-48, -28)
  point P1208 (-48, -28)
  point P1209 (-47, -8.6603)
  point P1210 (-48, -28)
  point P1211 (-64, -17.3205)
  point P1212 (-48, -28)
  point P1213 (-48, -28)
  point P1214 (-48, -28)
  point P1215 (-48, -28)
  point P1216 (0, -17.3205)
  point P1217 (-64, -17.3205)
  point P1218 (-16, -28)
  point P1219 (16, -28)
  point P1220 (16, -28)
  point P1221 (16, -28)
  point P1222 (0, -17.3205)
  point P1223 (-16, -28)
  point P1224 (-64, -17.3205)
  point P1225 (-48, -28)
  point P1226 (-48, -28)
  point P1227 (16, -28)
  point P1228 (16, -28)
  point P1229 (0, -17.3205)
  point P1230 (16, -28)
  point P1231 (-16, -28)
  point P1232 (-16, -28)
  point P1233 (32, -17.3205)
  point P1234 (-16, -28)
  point P1235 (16, -28)
  point P1236 (-48, -28)
  point P1237 (16, -28)
  point P1238 (16, -28)
  point P1239 (-16, -28)
  point P1240 (16, -28)
  point P1241 (16, -28)
  point P1242 (-16, -28)
  point P1243 (79, -8.6603)
  point P1244 (-49, -8.6603)
  point P1245 (-32, -17.3205)
  point P1246 (-16, -28)
  point P1247 (-16, -28)
  point P1248 (-16, -28)
  point P1249 (-79, -8.6603)
  point P1250 (-16, -28)
  point P1251 (49, -8.6603)
  point P1252 (-16, -28)
  point P1253 (-47, -8.6603)
  point P1254 (16, -28)
  point P1255 (-48, -28)
  point P1256 (-48, -28)
  point P1257 (-49, -8.6603)
  point P1258 (16, 28)
  point P1259 (-16, 28)
  point P1260 (-31, 19.3397)
  point P1261 (16, 28)
  point P1262 (-31, 19.3397)
  point P1263 (16, 28)
  point P1264 (-1, 19.3397)
  point P1265 (-48, 28)
  point P1266 (16, 28)
  point P1267 (64, 17.3205)
  point P1268 (-1, 19.3397)
  point P1269 (16, 28)
  point P1270 (33, 19.3397)
  point P1271 (31, 19.3397)
  point P1272 (-64, 17.3205)
  point P1273 (-16, 28)
  point P1274 (-16, 28)
  point P1275 (-16, 28)
  point P1276 (64, 17.3205)
  point P1277 (-16, 28)
  point P1278 (-64, 17.3205)
  point P1279 (16, 28)
  point P1280 (-16, 28)
  point P1281 (-32, 17.3205)
  point P1282 (16, 28)
  point P1283 (63, 19.3397)
  point P1284 (33, 19.3397)
  point P1285 (31, 19.3397)
  point P1286 (16, 28)
  point P1287 (1, 19.3397)
  point P1288 (16, 28)
  point P1289 (16, 28)
  point P1290 (-16, 28)
  point P1291 (-16, 28)
  point P1292 (-16, 28)
  point P1293 (-32, 17.3205)
  point P1294 (32, 17.3205)
  point P1295 (0, 17.3205)
  point P1296 (-16, 28)
  point P1297 (16, 28)
  point P1298 (-48, 28)
  point P1299 (-31, 19.3397)
  point P1300 (-48, 28)
  point P1301 (0, 17.3205)
  point P1302 (16, 28)
  point P1303 (-16, 28)
  point P1304 (-16, 28)
  point P1305 (-16, 28)
  point P1306 (16, 28)
  point P1307 (1, 19.3397)
  point P1308 (-32, 17.3205)
  point P1309 (-16, 28)
  point P1310 (32, 17.3205)
  point P1311 (16, 28)
  point P1312 (-32, 17.3205)
  point P1313 (-1, 19.3397)
  point P1314 (32, 17.3205)
  point P1315 (1, 19.3397)
  point P1316 (31, 19.3397)
  point P1317 (16, 28)
  point P1318 (-16, 28)
  point P1319 (16, 28)
  point P1320 (16, 28)
  point P1321 (16, 28)
  point P1322 (31, 19.3397)
  point P1323 (0, 17.3205)
  point P1324 (-1, 19.3397)
  point P1325 (16, 28)
  point P1326 (16, 28)
  point P1327 (-16, 28)
  point P1328 (-31, 19.3397)
  point P1329 (-31, 19.3397)
  point P1330 (16, 28)
  point P1331 (-1, 19.3397)
  point P1332 (-1, 19.3397)
  point P1333 (-32, 17.3205)
  point P1334 (-16, 28)
  point P1335 (32, 17.3205)
  point P1336 (-16, 28)
  point P1337 (16, 28)
  point P1338 (0, 17.3205)
  point P1339 (-16, 28)
  point P1340 (-48, 28)
  point P1341 (-31, 19.3397)
  point P1342 (31, 19.3397)
  point P1343 (63, 19.3397)
  point P1344 (-63, 19.3397)
  point P1345 (-48, 28)
  point P1346 (-48, 28)
  point P1347 (-48, 28)
  point P1348 (33, 19.3397)
  point P1349 (-48, 28)
  point P1350 (-32, 17.3205)
  point P1351 (-33, 19.3397)
  point P1352 (-48, 28)
  point P1353 (-48, 28)
  point P1354 (63, 19.3397)
  point P1355 (-33, 19.3397)
  point P1356 (-16, 28)
  point P1357 (-16, 28)
  point P1358 (-63, 19.3397)
  point P1359 (32, 17.3205)
  point P1360 (0, 17.3205)
  point P1361 (-16, 28)
  point P1362 (1, 19.3397)
  point P1363 (-48, 28)
  point P1364 (-33, 19.3397)
  point P1365 (-63, 19.3397)
  point P1366 (1, 19.3397)
  point P1367 (-33, 19.3397)
  point P1368 (-48, 28)
  point P1369 (16, 28)
  point P1370 (-16, 28)
  point P1371 (16, 28)
  point P1372 (-48, 28)
  point P1373 (-48, 28)
  point P1374 (-48, 28)
  point P1375 (-31, 19.3397)
  point P1376 (-16, 28)
  point P1377 (1, 19.3397)
  point P1378 (31, 19.3397)
  point P1379 (31, 19.3397)
  point P1380 (64, 0)
  point P1381 (-64, 0)
  point P1382 (-32, -17.3205)
  point P1383 (64, 0)
  point P1384 (-64, 0)
  point P1385 (64, 0)
  point P1386 (-47, -8.6603)
  point P1387 (-49, -8.6603)
  point P1388 (0, -17.3205)
  point P1389 (-64, -17.3205)
  point P1390 (-64, 0)
  point P1391 (-47, -8.6603)
  point P1392 (-49, -8.6603)
  point P1393 (64, 0)
  point P1394 (-64, -17.3205)
  point P1395 (64, 0)
  point P1396 (33, -19.3397)
  point P1397 (32, -17.3205)
  point P1398 (0, -17.3205)
  point P1399 (0, -17.3205)
  point P1400 (-33, 19.3397)
  point P1401 (-48, 28)
  point P1402 (-48, 28)
  point P1403 (-16, 28)
  point P1404 (1, 19.3397)
  point P1405 (1, 19.3397)
  point P1406 (-31, 19.3397)
  point P1407 (-48, 28)
  point P1408 (0, 17.3205)
  point P1409 (16, 28)
  point P1410 (-63, 19.3397)
  point P1411 (-16, 28)
  point P1412 (31, 19.3397)
  point P1413 (-33, 19.3397)
  point P1414 (16, 28)
  point P1415 (-33, 19.3397)
  point P1416 (63, 19.3397)
  point P1417 (1, 19.3397)
  point P1418 (-48, 28)
  point P1419 (-63, 19.3397)
  point P1420 (-64, 17.3205)
  point P1421 (-64, 17.3205)
  point P1422 (16, 28)
  point P1423 (-48, 28)
  point P1424 (-48, 28)
  point P1425 (16, 28)
  point P1426 (-48, 28)
  point P1427 (-1, 19.3397)
  point P1428 (-63, 19.3397)
  point P1429 (-48, 28)
  point P1430 (64, 17.3205)
  point P1431 (-1, 19.3397)
  point P1432 (-1, 19.3397)
  point P1433 (-63, 19.3397)
  point P1434 (-48, 28)
  point P1435 (64, 17.3205)
  point P1436 (33, 19.3397)
  point P1437 (16, 28)
  point P1438 (-16, 28)
  point P1439 (16, 28)
  point P1440 (1, 19.3397)
  point P1441 (-16, 28)
  point P1442 (16, 28)
  point P1443 (16, 28)